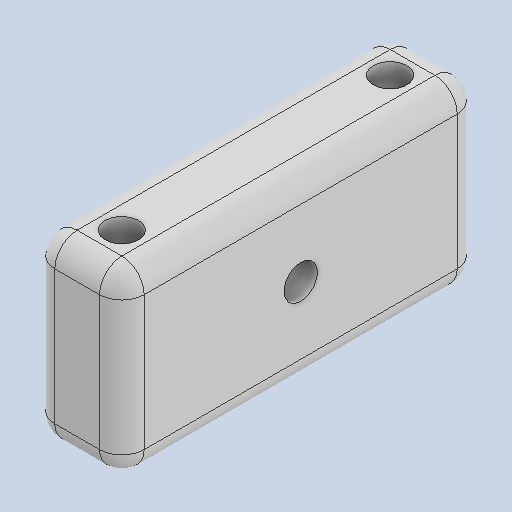
# Autodesk Inventor part: piston connection
Saved by Autodesk Inventor 2023 (Build 270158000, 158)
## iProperties
Created: 2023-01-25
Part Number: piston connection
Material: Generic
Document SubType Name: Modeling
Designer: Gabriel - T3 CAD
Density: 1 g/cm^3
Appearance: Default
Mass: 14.5295 g
Surface Area: 48.6331 cm^2
Volume: 14.5295 cm^3
Author: Gabriel - T3 CAD
Autodesk Inventor part; units mm, degrees
ref_plane "YZ Plane" through (0, 0, 0) normal (1, 0, 0) x (0, 1, 0)
ref_plane "XZ Plane" through (0, 0, 0) normal (0, 1, 0) x (-1, 0, 0)
ref_plane "XY Plane" through (0, 0, 0) normal (0, 0, 1) x (1, 0, 0)
sketch "Sketch1" plane through (0, 0, 0) normal (0, 1, 0) x (-1, 0, 0)
  line L0 (0, 0) -> (12.7, 0)
  line L1 (12.7, 0) -> (12.7, 50.8)
  line L2 (12.7, 50.8) -> (0, 50.8)
  line L3 (0, 50.8) -> (0, 0)
  circle A0 centre (6.35, 6.35) radius 2.3813
  circle A1 centre (6.35, 44.45) radius 2.3813
  dimension "d0" = 12.7
  dimension "d1" = 50.8
  dimension "d2" = 6.35
  dimension "d3" = 6.35
  dimension "d4" = 4.7625
  dimension "d5" = 6.35
  dimension "d6" = 4.7625
  dimension "d7" = 6.35
  constraints: 8 end point, 2 centre point, 2 parallel, 1 horizontal, 1 perpendicular
  measures "d0" distance of L2.end L1.end
  measures "d1" distance of L1.end L0.end
  measures "d2" distance from line of L0 A0.centre
  measures "d3" distance from line of L1 A0.centre
  measures "d4" diameter of A0
  measures "d5" distance from line of L1 A1.centre
  measures "d6" diameter of A1
  measures "d7" distance from line of L2 A1.centre
extrude "Extrusion1" add sketch "Sketch1" along normal blind 25.4
sketch "Sketch4" plane through (0, 0, 50.8) normal (1, 0, 0) x (0, 0, -1)
  circle A0 centre (25.4, 12.7) radius 2.3813
  line L0 (0, 0) -> (0, 25.4) projected
  line L1 (0, 0) -> (50.8, 0) projected
  dimension "d30" = 25.4
  dimension "d31" = 12.7
  dimension "d32" = 4.7625
  constraints: 1 centre point
  measures "d30" distance from line of L0 A0.centre
  measures "d31" distance from line of L1 A0.centre
  measures "d32" diameter of A0
extrude "Extrusion4" cut sketch "Sketch4" against normal blind 25.4
fillet "Fillet1" radius 3.175 4 edges at (-12.7, 25.4, 25.4) (0, 25.4, 25.4) (0, 0, 25.4) (-12.7, 0, 25.4)
fillet "Fillet2" radius 3.175 16 edges at (-0.9299, 24.4701, 50.8) (-6.35, 25.4, 50.8) (-11.7701, 24.4701, 50.8) (-12.7, 12.7, 50.8) (-11.7701, 0.9299, 50.8) (-6.35, 0, 50.8) (-0.9299, 0.9299, 50.8) (0, 12.7, 50.8) (-0.9299, 24.4701, 0) (-6.35, 25.4, 0) (-11.7701, 24.4701, 0) (-12.7, 12.7, 0) (-11.7701, 0.9299, 0) (-6.35, 0, 0) (-0.9299, 0.9299, 0) (0, 12.7, 0)
body "Solid1"
